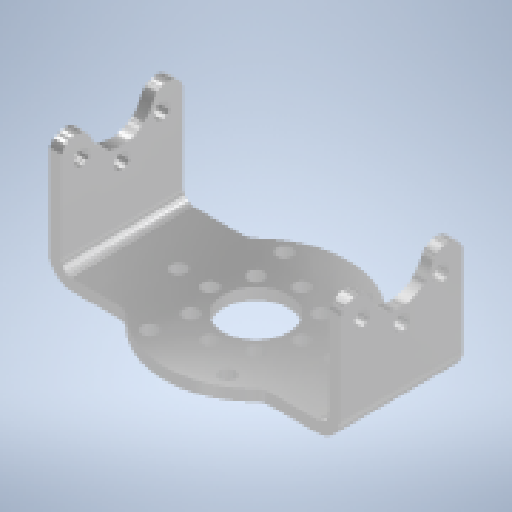
# Autodesk Inventor part: sholder
Saved by Autodesk Inventor 2024.1 (Build 281209000, 209)
## iProperties
Created: 2024-02-14
Part Number: sholder
Material: アルミニウム 6061
Document SubType Name: Sheet Metal
Designer: hibik
Density: 2.7 g/cm^3
Sheet Metal Rule: Default_mm
Appearance: アルミニウム - フラット
Author: hibik
Autodesk Inventor part; units mm, degrees
ref_plane "YZ Plane" through (0, 0, 0) normal (1, 0, 0) x (0, 1, 0)
ref_plane "XZ Plane" through (0, 0, 0) normal (0, 1, 0) x (-1, 0, 0)
ref_plane "XY Plane" through (0, 0, 0) normal (0, 0, 1) x (1, 0, 0)
sketch "スケッチ1" plane through (0, 0, 0) normal (0, 1, 0) x (-1, 0, 0)
  line L0 (19, 8) -> (-19, 8)
  line L1 (-19, 8) -> (-19, -8)
  line L2 (-19, -8) -> (19, -8)
  line L3 (19, -8) -> (19, 8)
  line L4 (19, 8) -> (-19, -8) construction
  line L5 (-19, 8) -> (19, -8) construction
  circle A0 centre (0, 0) radius 4.25
  circle A1 centre (0, 0) radius 6
  circle A2 centre (0, 6) radius 1
  line L6 (0, -16.8) -> (0, 16.8)
  circle A3 centre (-4.2426, 4.2426) radius 1
  circle A4 centre (-6, 0) radius 1
  circle A5 centre (-4.2426, -4.2426) radius 1
  circle A6 centre (0, -6) radius 1
  circle A7 centre (4.2426, -4.2426) radius 1
  circle A8 centre (0, 0) radius 12
  circle A9 centre (6, 0) radius 1
  circle A10 centre (4.2426, 4.2426) radius 1
  point P0 (-8.9443, -8)
  point P1 (8.9443, -8)
  point P2 (-8.9443, 8)
  point P3 (8.9443, 8)
  dimension "d1" = 12
  dimension "d0" = 8.5
  dimension "d2" = 2
  dimension "d5" = 360
  dimension "d8" = 16
  dimension "d9" = 38
  dimension "d21" = 24
  measures "d0" diameter of A0
  measures "d2" diameter of A2
  measures "d8" distance of L2.end L0.start
  measures "d9" distance of L0.start L0.end
  measures "d21" diameter of A8
extrude "プレート1" add sketch "スケッチ1" along normal blind 1.5 contours L3 L2 A8 L0 | A8 L2 L6 A6 A1 A7 A9 A10 A2 L0 | L0 L6 A8 | L6 A2 A1 A3 A4 A5 A6 L2 A8 L0 | L0 A8 L6 | A8 L6 L2 | A8 L2 L1 L0 | L6 A8 L2 | A2 L6 A0 A6 A1 A5 A4 A3 | A1 A10 A9 A7 A6 L6 A0 A2
sketch "スケッチ2" plane through (-17.5, 0, 8) normal (-1, 0, 0) x (0, -1, 0)
  line L0 (0, -16) -> (0, 0)
  line L1 (0, 0) -> (-20, 0)
  line L2 (-20, 0) -> (-20, -16)
  line L3 (-20, -16) -> (0, -16)
  constraints: 6 end point, 1 horizontal, 1 perpendicular, 1 vertical
edge flange "フランジ1" height 20 angle 90 thickness 1.5 bend radius 1.5 thickness toward (-1, 0, 0) relief straight relief width 1.5 relief depth 0.75 corner gap 1.5 corner form 0 edges at (-19, 1.5, 0) (19, 1.5, 0) wall of the first edge with corners at (-17.5, 0, -8) (-17.5, 0, 8) (-17.5, 20, 8) (-17.5, 20, -8)
bend "曲げ1"
corner "コーナー1"
sketch "スケッチ3" plane through (0, 1.5, 0) normal (0, 1, 0) x (1, 0, 0)
  circle A0 centre (8.7685, -5.0625) radius 1 projected
  circle A1 centre (8.7685, 5.0625) radius 1 projected
  circle A2 centre (0, 10.125) radius 1 projected
  circle A3 centre (-8.7685, 5.0625) radius 1 projected
  circle A4 centre (-8.7685, -5.0625) radius 1 projected
  circle A5 centre (0, -10.125) radius 1 projected
  point P0 (0, 0)
extrude "切り取り1" cut sketch "スケッチ3" against normal blind 1.5
sketch "スケッチ4" plane through (19, 20, 8) normal (1, 0, 0) x (0, 0, -1)
  circle A0 centre (8, -4) radius 4.25
  line L0 (0, -17) -> (16, -17) projected
  circle A1 centre (8, -4) radius 6 construction
  circle A2 centre (8, -10) radius 1
  circle A3 centre (12.2426, -8.2426) radius 1
  circle A4 centre (14, -4) radius 1
  circle A5 centre (12.2426, 0.2426) radius 1
  circle A6 centre (8, 2) radius 1
  circle A7 centre (3.7574, 0.2426) radius 1
  line L1 (16, -17) -> (16, 0) projected
  line L2 (0, 0) -> (16, 0)
  line L3 (16, 0) -> (16, -4)
  line L4 (16, -4) -> (0, -4)
  line L5 (0, -4) -> (0, 0)
  line L6 (0, 0) -> (16, 0) projected
  circle A8 centre (2, -4) radius 1
  circle A9 centre (3.7574, -8.2426) radius 1
  line L7 (8, -4) -> (16, -0.6863)
  line L8 (8, -4) -> (0, -0.6863)
  line L9 (2, -4) -> (3.7574, 0.2426)
  line L10 (12.2426, 0.2426) -> (14, -4)
  point P0 (8, -20)
  point P1 (8, -17)
  point P2 (8, -17)
  point P3 (13.1213, -1.8787)
  point P4 (2.8787, -1.8787)
  dimension "d24" = 13
  dimension "d25" = 8.5
  dimension "d26" = 12
  dimension "d27" = 2
  dimension "d30" = 360
  constraints: 16 end point, 10 centre point, 5 midpoint, 5 point on line, 4 coincident, 2 parallel, 2 point on circle, 2 vertical alignment, 1 collinear, 1 horizontal, 1 perpendicular, 23 other
  measures "d24" distance from line of L0 A0.centre
  measures "d25" diameter of A0
  measures "d26" diameter of A1
  measures "d27" diameter of A2
extrude "切り取り2" cut sketch "スケッチ4" against normal blind 38 contours L4 L7 A0 | A0 L4 | L7 L8 A0 L2 | A0 L2 A5 L10 L7 | A0 L8 L4 | L4 A4 | A4 L10 L4 | L2 A0 | L10 A5 L2 L1 L7 | L8 L9 A7 L2 A0 | A8 L4 | L4 L9 A8 | A4 L4 L10 | L2 L10 A5 | L10 L2 A5 | L8 L5 L2 A7 L9 | L4 A8 L9 | L2 A7 | A7 L9 L2 | A7 L2 L9 | A2 | A3 | A9
fillet "フィレット1" radius 2 12 edges at (-8.9443, 0.75, 8) (8.9443, 0.75, 8) (8.9443, 0.75, -8) (-8.9443, 0.75, -8) (18.25, 17.6264, 3.9265) (18.25, 17.6264, -3.9265) (-18.25, 17.6264, 3.9265) (-18.25, 17.6264, -3.9265) (18.25, 19.3137, 8) (18.25, 19.3137, -8) (-18.25, 19.3137, -8) (-18.25, 19.3137, 8)
equation "\"d22\" = Thickness"
equation "\"d10\" = Thickness"
equation "\"d11\" = BendReliefWidth"
equation "\"d12\" = BendReliefDepth"
equation "\"d13\" = MinimumRemnant"
equation "\"d14\" = TransitionRadius"
equation "\"d17\" = BendRadius"
equation "\"d18\" = CornerReliefSize"
equation "\"d19\" = GapSize"
equation "\"d20\" = JacobiRadiusSize"
equation "\"BendRadius\" = Thickness"
equation "\"BendReliefWidth\" = Thickness"
equation "\"BendReliefDepth\" = 0.5 * Thickness"
equation "\"CornerReliefSize\" = 4 * Thickness"
equation "\"MinimumRemnant\" = 2 * Thickness"
equation "\"TransitionRadius\" = BendRadius"
equation "\"JacobiRadiusSize\" = BendRadius"
equation "\"GapSize\" = Thickness"
equation "\"Thickness\" = 1.5"
